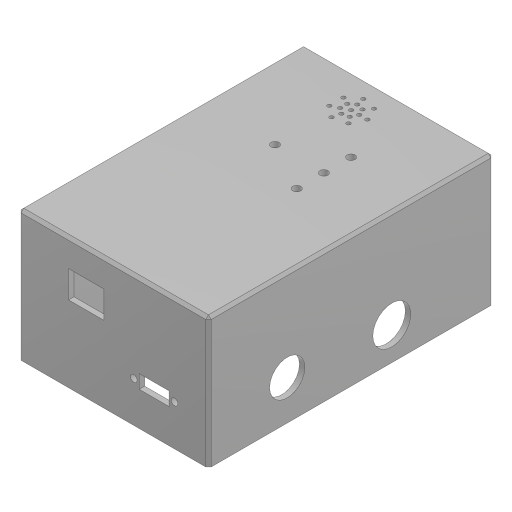
# Autodesk Inventor part: Top
Saved by Autodesk Inventor 2023.1 (Build 271208000, 208)
## iProperties
Created: 2022-08-29
Part Number: Top
Material: PC/ABS-Kunststoff
Document SubType Name: Modeling
Designer: tland
Density: 0.357273 g/cm^3
Appearance: Glatt - Mittelgrau
Author: tland
Autodesk Inventor part; units mm, degrees
note: some values were not read from the file. Chosen so that the rebuilt part matches the saved one: direction of "Sensor"; direction of "Switch".
ref_plane "YZ Plane" through (0, 0, 0) normal (1, 0, 0) x (0, 1, 0)
ref_plane "XZ Plane" through (0, 0, 0) normal (0, 1, 0) x (-1, 0, 0)
ref_plane "XY Plane" through (0, 0, 0) normal (0, 0, 1) x (1, 0, 0)
sketch "Skizze1" plane through (0, 0, 0) normal (0, 1, 0) x (-1, 0, 0)
  line L0 (35, 52.5) -> (-35, 52.5)
  line L1 (-35, 52.5) -> (-35, -52.5)
  line L2 (-35, -52.5) -> (35, -52.5)
  line L3 (35, -52.5) -> (35, 52.5)
  point P0 (0, 0)
  point P1 (0, 52.5)
  point P2 (35, 0)
  dimension "d0" = 105
  dimension "d1" = 70
  constraints: 8 end point, 2 midpoint, 2 parallel, 1 horizontal, 1 horizontal alignment, 1 perpendicular, 1 vertical alignment
  measures "d0" distance of L2.end L0.start
  measures "d1" distance of L0.start L0.end
extrude "Extrusion1" add sketch "Skizze1" along normal blind 48
shell "Wandung1" thickness 2 removed faces 1 at (11.6667, 0, 17.5)
sketch "Skizze25" plane through (0, 0, 0) normal (0, -1, 0) x (1, 0, 0)
  line L0 (33, 50.5) -> (33, -50.5) construction
  line L1 (-33, 50.5) -> (33, 50.5) construction
  line L2 (-33, -50.5) -> (-33, 50.5) construction
  line L3 (33, -50.5) -> (-33, -50.5) construction
  line L4 (33, 50.5) -> (28, 50.5)
  line L5 (28, 50.5) -> (28, 45.5)
  line L6 (28, 45.5) -> (33, 45.5)
  line L7 (33, 45.5) -> (33, 50.5)
  line L8 (33, -50.5) -> (28, -50.5)
  line L9 (28, -50.5) -> (28, -45.5)
  line L10 (28, -45.5) -> (33, -45.5)
  line L11 (33, -45.5) -> (33, -50.5)
  line L12 (-33, 50.5) -> (-28, 50.5)
  line L13 (-28, 50.5) -> (-28, 45.5)
  line L14 (-28, 45.5) -> (-33, 45.5)
  line L15 (-33, 45.5) -> (-33, 50.5)
  line L16 (-33, -50.5) -> (-28, -50.5)
  line L17 (-28, -50.5) -> (-28, -45.5)
  line L18 (-28, -45.5) -> (-33, -45.5)
  line L19 (-33, -45.5) -> (-33, -50.5)
  point P0 (0, 0)
  dimension "d208" = 5
  dimension "d209" = 5
  constraints: 32 end point, 8 parallel, 6 equal length, 4 horizontal, 4 perpendicular
  measures "d208" distance of L6.end L5.end
  measures "d209" distance of L4.end L5.end
extrude "Extrusion12" add sketch "Skizze25" against normal blind 8
chamfer "Fase2" distance 5 angle 45 2 edges at (30.5, 8, 45.5) (28, 8, 48)
chamfer "Fase3" distance 5 angle 45 2 edges at (30.5, 8, -45.5) (28, 8, -48)
chamfer "Fase4" distance 5 angle 45 2 edges at (-28, 8, 48) (-30.5, 8, 45.5)
chamfer "Fase5" distance 5 angle 45 2 edges at (-28, 8, -48) (-30.5, 8, -45.5)
sketch "Skizze26" plane through (0, 0, 0) normal (0, -1, 0) x (1, 0, 0)
  line L0 (-31, 48.5) -> (31, 48.5) construction
  line L1 (31, 48.5) -> (31, -48.5) construction
  line L2 (31, -48.5) -> (-31, -48.5) construction
  line L3 (-31, -48.5) -> (-31, 48.5) construction
  point P0 (0, 0)
  point P1 (-31, 0)
  point P2 (0, 48.5)
  dimension "d224" = 97
  dimension "d225" = 62
  constraints: 8 end point, 4 coincident, 2 midpoint, 2 parallel, 1 horizontal, 1 horizontal alignment, 1 perpendicular, 1 vertical alignment
  measures "d224" distance of L2.end L0.start
  measures "d225" distance of L0.start L0.end
hole "Bohrung14" at (-31, 0, 48.5) at (31, 0, 48.5) at (31, 0, -48.5) at (-31, 0, -48.5) direction (0, 1, 0) diameter 2.8 depth 8
chamfer "Fase6" distance 1 angle 45 8 edges at (0, 48, -52.5) (35, 48, 0) (35, 24, -52.5) (0, 48, 52.5) (35, 24, 52.5) (-35, 24, 52.5) (-35, 48, 0) (-35, 24, -52.5)
sketch "Skizze11" plane through (35, 45, -52.5) normal (1, 0, 0) x (0, 0, 1)
  circle A0 centre (37.5, 33) radius 9 construction
  line L0 (104, 45) -> (1, 45) construction
  point P0 (52.5, 45)
  point P1 (52.5, 45)
  point P2 (52.5, 45)
  dimension "d238" = 18
  dimension "d285" = 15
  dimension "d286" = 12
  constraints: 2 midpoint, 1 centre point, 1 coincident
  measures "d238" diameter of A0
  measures "d285" horizontal distance of A0.centre point (52.5, 45)
  measures "d286" vertical distance of point (52.5, 45) A0.centre
hole "Button" at (35, 12, -15) direction (-1, 0, 0) diameter 14 depth 5 tip angle 118
sketch "Skizze12" plane through (0, 48, 0) normal (0, 1, 0) x (1, 0, 0)
  point P0 (0, 0)
  point P1 (10, 25)
  point P2 (10, 15)
  point P3 (10, 5)
  dimension "d239" = 5
  dimension "d240" = 10
  dimension "d241" = 10
  dimension "d258" = 10
  constraints: 2 vertical alignment
  measures "d239" vertical distance of point (10, 5) point (0, 0)
  measures "d240" distance of point (10, 15) point (10, 5)
  measures "d241" distance of point (10, 15) point (10, 25)
  measures "d258" horizontal distance of point (0, 0) point (10, 5)
hole "LEDS" at (10, 48, -25) at (10, 48, -15) at (10, 48, -5) direction (0, -1, 0) diameter 3 end through all
sketch "Skizze14" plane through (29, 0, -52.5) normal (0, 0, -1) x (-1, 0, 0)
  line L0 (-5, 0) -> (63, 0) construction
  point P0 (9, 10)
  point P1 (29, 0)
  point P2 (29, 0)
  point P3 (29, 0)
  point P4 (29, 0)
  dimension "d268" = 10
  dimension "d287" = 20
  constraints: 3 midpoint
  measures "d268" vertical distance of point (29, 0) point (9, 10)
  measures "d287" horizontal distance of point (9, 10) point (29, 0)
hole "Sensor" at (20, 10, -52.5) direction (0, 0, 1) diameter 8 end up to surface
sketch "Skizze28" plane through (-33, 46, -50.5) normal (0, 0, 1) x (1, 0, 0)
  circle A0 centre (53, -36) radius 4 construction
  line L0 (60.5, -43.5) -> (45.5, -43.5)
  line L1 (45.5, -43.5) -> (45.5, -28.5)
  line L2 (45.5, -28.5) -> (60.5, -28.5)
  line L3 (60.5, -28.5) -> (60.5, -43.5)
  point P0 (33, -46)
  point P1 (53, -43.5)
  point P2 (60.5, -36)
  dimension "d261" = 15
  constraints: 8 end point, 2 midpoint, 2 parallel, 2 perpendicular, 1 horizontal, 1 horizontal alignment, 1 vertical alignment
  measures "d261" distance of L0.start L0.end
extrude "Extrusion14" cut sketch "Skizze28" against normal blind 0.5
sketch "Skizze20" plane through (-29, 0, 52.5) normal (0, 0, 1) x (1, 0, 0)
  line L0 (38.5, 17.5) -> (49.5, 17.5)
  line L1 (49.5, 17.5) -> (49.5, 12.5)
  line L2 (49.5, 12.5) -> (38.5, 12.5)
  line L3 (38.5, 12.5) -> (38.5, 17.5)
  line L4 (38.5, 15) -> (49.5, 15) construction
  line L5 (44, 17.5) -> (44, 12.5) construction
  line L6 (-5, 0) -> (63, 0) construction
  point P0 (51.5, 15)
  point P1 (36.5, 15)
  point P2 (44, 15)
  point P3 (29, 0)
  point P4 (29, 0)
  point P5 (29, 0)
  point P6 (44, 15)
  point P7 (29, 0)
  dimension "d149" = 11
  dimension "d150" = 5
  dimension "d153" = 15
  dimension "d249" = 15
  dimension "d259" = 15
  constraints: 12 end point, 9 midpoint, 2 parallel, 1 horizontal, 1 horizontal alignment, 1 perpendicular, 1 point on line, 1 symmetric about line
  measures "d149" distance of L0.start L0.end
  measures "d150" distance of L2.end L0.start
  measures "d153" distance of point (51.5, 15) point (36.5, 15)
  measures "d249" horizontal distance of point (29, 0) point (44, 15)
  measures "d259" horizontal distance of point (44, 15) point (29, 0)
extrude "Extrusion9" cut sketch "Skizze20" against normal up to surface (2 mm away)
hole "Switch" at (7.5, 15, 52.5) at (22.5, 15, 52.5) direction (0, 0, -1) diameter 2.5 depth 2
sketch "Skizze22" plane through (35, 0, 52.5) normal (-1, 0, 0) x (0, 0, 1)
  line L0 (-104, 0) -> (-1, 0) construction
  point P0 (-29, 14.5)
  point P1 (-52.5, 0)
  point P2 (-52.5, 0)
  point P3 (-52.5, 0)
  point P4 (0, 0)
  dimension "d250" = 23.5
  dimension "d251" = 14.5
  dimension "d260" = 29
  constraints: 2 midpoint
  measures "d250" horizontal distance of point (-52.5, 0) point (-29, 14.5)
  measures "d251" vertical distance of point (-29, 14.5) point (-52.5, 0)
  measures "d260" horizontal distance of point (-29, 14.5) point (0, 0)
hole "nRF-Antenna" at (35, 14.5, 23.5) direction (-1, 0, 0) diameter 13 depth 8 tip angle 118
sketch "Skizze27" plane through (-33, 46, 50.5) normal (0, -1, 0) x (1, 0, 0)
  line L0 (59, -94) -> (7, -94) construction
  line L1 (7, -94) -> (7, -7) construction
  line L2 (7, -7) -> (59, -7) construction
  line L3 (59, -7) -> (59, -94) construction
  circle A0 centre (59, -94) radius 3.5
  circle A1 centre (7, -94) radius 3.5
  circle A2 centre (7, -7) radius 3.5
  circle A3 centre (59, -7) radius 3.5
  circle A4 centre (59, -94) radius 1.4
  circle A5 centre (7, -94) radius 1.4
  circle A6 centre (59, -7) radius 1.4
  circle A7 centre (7, -7) radius 1.4
  point P0 (33, -50.5)
  point P1 (59, -50.5)
  point P2 (33, -94)
  dimension "d252" = 7
  dimension "d253" = 87
  dimension "d254" = 52
  dimension "d255" = 2.8
  constraints: 8 centre point, 8 coincident, 8 end point, 6 equal radius, 2 midpoint, 2 parallel, 1 horizontal, 1 horizontal alignment, 1 perpendicular, 1 vertical alignment
  measures "d252" diameter of A0
  measures "d253" distance of L2.end L0.start
  measures "d254" distance of L0.start L0.end
  measures "d255" diameter of A4
extrude "PCB-holder" add sketch "Skizze27" along normal blind 10
sketch "Skizze29" plane through (0, 48, 0) normal (0, 1, 0) x (1, 0, 0)
  point P0 (0, 0)
  point P1 (-8, 15)
  dimension "d269" = 8
  dimension "d278" = 15
  measures "d269" horizontal distance of point (0, 0) point (-8, 15)
  measures "d278" vertical distance of point (-8, 15) point (0, 0)
hole "LED Green" at (-8, 48, -15) direction (0, -1, 0) diameter 3 depth 8 tip angle 118
sketch "Skizze30" plane through (34, 0, -52.5) normal (0, 0, -1) x (-1, 0, 0)
  line L0 (16.5, 17) -> (31.5, 17)
  line L1 (31.5, 17) -> (31.5, 28)
  line L2 (31.5, 28) -> (16.5, 28)
  line L3 (16.5, 28) -> (16.5, 17)
  line L4 (24, 17) -> (24, 28) construction
  line L5 (16.5, 22.5) -> (31.5, 22.5) construction
  line L6 (0, 0) -> (68, 0) construction
  line L7 (40.5, 48) -> (43.5, 48) construction
  line L8 (22.5, 48) -> (25.5, 48) construction
  line L9 (22.5, 48) -> (25.5, 48) construction
  line L10 (22.5, 48) -> (25.5, 48) construction
  line L11 (0, 48) -> (68, 48) construction
  line L12 (68, 48) -> (0, 48) construction
  point P0 (34, 0)
  point P1 (34, 0)
  point P2 (24, 22.5)
  point P3 (34, 0)
  dimension "d279" = 15
  dimension "d280" = 11
  dimension "d282" = 10
  dimension "d288" = 20
  constraints: 12 end point, 7 midpoint, 2 parallel, 1 horizontal, 1 perpendicular
  measures "d279" distance of L0.start L0.end
  measures "d280" distance of L2.end L0.start
  measures "d282" horizontal distance of point (34, 0) L4.start
  measures "d288" distance between parallel lines of L2 L12
extrude "Arduino Programming" [suppressed]
sketch "Skizze31" plane through (-34, 0, 52.5) normal (0, 0, 1) x (1, 0, 0)
  line L0 (17.5, 28) -> (30.5, 28)
  line L1 (30.5, 28) -> (30.5, 38)
  line L2 (30.5, 38) -> (17.5, 38)
  line L3 (17.5, 38) -> (17.5, 28)
  line L4 (24, 28) -> (24, 38) construction
  line L5 (17.5, 33) -> (30.5, 33) construction
  line L6 (0, 0) -> (68, 0) construction
  point P0 (34, 0)
  point P1 (34, 0)
  point P2 (24, 33)
  dimension "d289" = 10
  dimension "d290" = 33
  dimension "d291" = 13
  dimension "d292" = 10
  constraints: 12 end point, 6 midpoint, 2 parallel, 1 horizontal, 1 perpendicular
  measures "d289" distance from line of point (34, 0) L4
  measures "d290" vertical distance of point (34, 0) point (24, 33)
  measures "d291" distance of L0.start L0.end
  measures "d292" distance of L2.end L0.start
extrude "USB-C" cut sketch "Skizze31" against normal blind 10
sketch "Skizze32" plane through (0, 48, 0) normal (0, 1, 0) x (1, 0, 0)
  line L0 (34, 52.5) -> (-34, 52.5) construction
  point P0 (0, 0)
  point P1 (-5, 40)
  point P2 (-2, 40)
  point P3 (1, 40)
  dimension "d295" = 3
  dimension "d296" = 3
  dimension "d297" = 40
  dimension "d298" = 5
  dimension "d309" = 12.5
  constraints: 2 horizontal alignment
  measures "d295" distance of point (-2, 40) point (-5, 40)
  measures "d296" distance of point (1, 40) point (-2, 40)
  measures "d297" vertical distance of point (-5, 40) point (0, 0)
  measures "d298" horizontal distance of point (0, 0) point (-5, 40)
  measures "d309" distance from line of L0 point (-5, 40)
hole "Bohrung16" at (-5, 48, -40) at (-2, 48, -40) at (1, 48, -40) direction (0, -1, 0) diameter 1.5 depth 8 tip angle 118
pattern_circular "Runde Anordnung3" count 7 over 360 about axis through (-5, 44, -40) along (0, 1, 0) of "Bohrung16"
equation "\"d209\" = d208"
